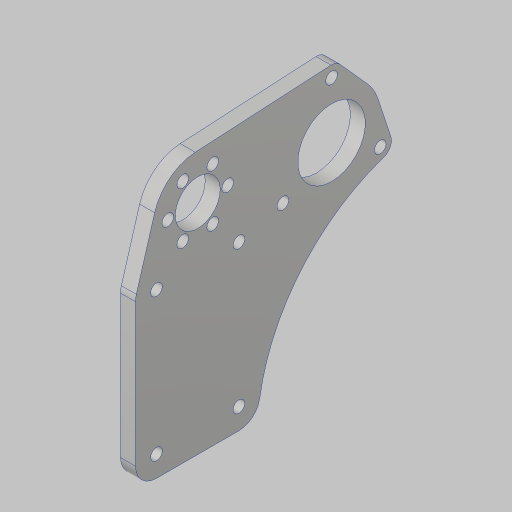
# Autodesk Inventor part: EL2-A-011
Saved by Autodesk Inventor 2023.5 (Build 275446000, 446)
## iProperties
Created: 2025-01-22
Part Number: EL2-A-011
Material: Aluminum 6061
Document SubType Name: Modeling
Designer: slick
Density: 2.7 g/cm^3
Appearance: Aluminum - Flat
Author: slick
Autodesk Inventor part; units mm, degrees
ref_plane "YZ Plane" through (0, 0, 0) normal (1, 0, 0) x (0, 1, 0)
ref_plane "XZ Plane" through (0, 0, 0) normal (0, 1, 0) x (-1, 0, 0)
ref_plane "XY Plane" through (0, 0, 0) normal (0, 0, 1) x (1, 0, 0)
sketch "Sketch1" plane through (0, 0, 0) normal (1, 0, 0) x (0, 1, 0)
  circle A0 centre (0, 0) radius 38.1 construction
  line L0 (27.94, -25.903) -> (27.94, -76.2) construction
  line L1 (27.94, -76.2) -> (-27.94, -76.2) construction
  line L2 (-27.94, -76.2) -> (-27.94, -25.903) construction
  line L3 (-30.1625, -17.4625) -> (30.1625, -17.4625) construction
  line L4 (30.1625, -17.4625) -> (30.1625, 17.4625) construction
  line L5 (30.1625, 17.4625) -> (-30.1625, 17.4625) construction
  line L6 (-30.1625, 17.4625) -> (-30.1625, -17.4625) construction
  line L7 (-30.1625, -17.4625) -> (30.1625, 17.4625) construction
  line L8 (30.1625, -17.4625) -> (-30.1625, 17.4625) construction
  circle A1 centre (30.1625, 17.4625) radius 2.5527 construction
  circle A2 centre (30.1625, -17.4625) radius 2.5527 construction
  circle A3 centre (-30.1625, -17.4625) radius 2.5527 construction
  circle A4 centre (-30.1625, 17.4625) radius 2.5527 construction
  point P0 (0, -76.2)
  dimension "d0" = 76.2
  dimension "d1" = 55.88
  dimension "d2" = 76.2
  dimension "d3" = 60.325
  dimension "d4" = 34.925
  dimension "d5" = 5.1054
  dimension "d6" = 5.1054
  dimension "d7" = 5.1054
  dimension "d8" = 5.1054
  constraints: 18 end point, 5 centre point, 5 coincident, 3 midpoint, 3 perpendicular, 2 parallel, 2 point on circle, 1 horizontal, 1 vertical, 1 vertical alignment
  measures "d0" diameter of A0
  measures "d1" distance of L0.end L1.end
  measures "d2" distance from line of point (0, 0) L1
  measures "d3" distance of L5.end L4.end
  measures "d4" distance of L4.end L3.end
  measures "d5" diameter of A1
  measures "d6" diameter of A2
  measures "d7" diameter of A3
  measures "d8" diameter of A4
sketch "Sketch2" plane through (0, 0, 0) normal (1, 0, 0) x (0, 1, 0)
  line L0 (-30.1625, -17.4625) -> (30.1625, -17.4625) construction
  circle A0 centre (30.1625, -17.4625) radius 2.5527 construction
  circle A1 centre (-30.1625, -17.4625) radius 2.5527 construction
  line L1 (-30.1625, 17.4625) -> (-30.1625, -17.4625) construction
  circle A2 centre (-30.1625, 17.4625) radius 2.5527 construction
  line L2 (30.1625, -17.4625) -> (30.1625, 17.4625) construction
  line L3 (30.1625, -17.4625) -> (-30.1625, 17.4625) construction
  line L4 (30.1625, 17.4625) -> (-30.1625, 17.4625) construction
  line L5 (-30.1625, -17.4625) -> (30.1625, 17.4625) construction
  circle A3 centre (30.1625, 17.4625) radius 2.5527 construction
  circle A4 centre (0, 0) radius 38.1 construction
  line L6 (27.94, -25.903) -> (27.94, -76.2) construction
  line L7 (27.94, -76.2) -> (-27.94, -76.2) construction
  line L8 (-27.94, -76.2) -> (-27.94, -25.903) construction
  circle A5 centre (53.34, 0) radius 12.7 construction
  circle A6 centre (46.99, -56.6939) radius 14.2875
  circle A7 centre (46.99, -56.6939) radius 30.5054 construction
  circle A8 centre (53.34, 0) radius 9.525
  circle A9 centre (53.34, 0) radius 19.05 construction
  circle A10 centre (46.99, -56.6939) radius 20.6375 construction
  circle A11 centre (30.1625, 17.4625) radius 8.9027 construction
  circle A12 centre (30.1625, -17.4625) radius 8.9027 construction
  circle A13 centre (-30.1625, -17.4625) radius 8.9027 construction
  circle A14 centre (-30.1625, 17.4625) radius 8.9027 construction
  line L9 (58.7594, 18.2629) -> (32.6952, 25.9973)
  line L10 (30.1625, 26.3652) -> (-30.1625, 26.3652)
  line L11 (-39.0652, 17.4625) -> (-39.0652, -17.4625)
  arc A15 (72.3606, 1.0578) -> (58.7594, 18.2629) centre (53.34, 0) ccw
  arc A16 (32.6952, 25.9973) -> (30.1625, 26.3652) centre (30.1625, 17.4625) ccw
  arc A17 (-30.1625, 26.3652) -> (-39.0652, 17.4625) centre (-30.1625, 17.4625) ccw
  arc A18 (-39.0652, -17.4625) -> (-31.5677, -26.2536) centre (-30.1625, -17.4625) ccw
  circle A19 centre (46.99, -56.6939) radius 23.8125 construction
  circle A20 centre (35.0838, -36.0717) radius 4.7625 construction
  circle A21 centre (35.0838, -77.3161) radius 4.7625 construction
  circle A22 centre (70.8025, -56.6939) radius 4.7625 construction
  line L12 (72.3606, 1.0578) -> (75.5577, -56.4294)
  arc A23 (73.9775, -60.2437) -> (75.5577, -56.4294) centre (70.8025, -56.6939) ccw
  arc A24 (30.4163, -78.263) -> (36.5704, -81.8406) centre (35.0838, -77.3161) ccw
  arc A25 (30.4163, -78.263) -> (-31.5677, -26.2536) centre (-43.9964, -104.0065) ccw
  line L13 (73.9775, -60.2437) -> (60.7483, -72.0762)
  line L14 (53.4323, -76.3001) -> (36.5704, -81.8406)
  arc A26 (53.4323, -76.3001) -> (60.7483, -72.0762) centre (46.99, -56.6939) ccw
  point P0 (0, -76.2)
  point P1 (64.3385, -6.35)
  point P2 (64.3385, 6.35)
  point P3 (53.34, 12.7)
  point P4 (42.3415, 6.35)
  point P5 (42.3415, -6.35)
  point P6 (53.34, -12.7)
  dimension "d9" = 25.4
  dimension "d10" = 25.4
  dimension "d11" = 76.2
  dimension "d14" = 360
  dimension "d16" = 28.575
  dimension "d17" = 57.0484
  dimension "d18" = 19.05
  dimension "d19" = 61.0108
  dimension "d20" = 19.05
  dimension "d21" = 6.35
  dimension "d22" = 6.35
  dimension "d23" = 6.35
  dimension "d40" = 9.525
  dimension "d43" = 360
  dimension "d45" = 9.525
  dimension "d46" = 9.525
  dimension "d47" = 9.525
  dimension "d48" = 78.74
  constraints: 30 point on circle, 20 centre point, 16 coincident, 12 end point, 12 tangent, 3 equal radius, 2 horizontal alignment, 1 horizontal, 1 vertical alignment, 17 other
  measures "d10" distance from line of L6 A9.centre
  measures "d11" distance from line of L7 A9.centre
  measures "d16" diameter of A6
  measures "d17" distance of A6.centre A9.centre
  measures "d18" distance from line of L6 A6.centre
  measures "d19" diameter of A7
  measures "d20" diameter of A8
  measures "d22" radial gap between concentric circles of A6 A10
  measures "d23" radial gap between concentric circles of A3 A11
  measures "d45" diameter of A20
  measures "d46" diameter of A21
  measures "d47" diameter of A22
  measures "d48" radius of A25
extrude "Extrusion1" add sketch "Sketch2" along normal blind 6.35
hole "Motor Mount Holes" at (0, -30.1625, -17.4625) at (0, 30.1625, -17.4625) at (0, -30.1625, 17.4625) at (0, 30.1625, 17.4625) at (0, 0, -76.2) at (0, 64.3385, -6.35) at (0, 64.3385, 6.35) at (0, 53.34, 12.7) at (0, 42.3415, 6.35) at (0, 42.3415, -6.35) at (0, 53.34, -12.7) direction (1, 0, 0) diameter 4.9784 end through all clearance for "Flat Head Machine Screw (82)" size "#10" standard "Ansi Unified Screw Threads"
hole "Hole3" at (0, 70.8025, -56.6939) at (0, 35.0838, -36.0717) at (0, 35.0838, -77.3161) direction (1, 0, 0) diameter 4.9784 end through all clearance for "Flat Head Machine Screw (82)" size "#10" standard "Ansi Unified Screw Threads"
body "Solid1"
